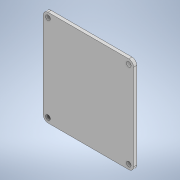
# Autodesk Inventor part: 视孔盖2
Saved by Autodesk Inventor 2020 (Build 240168000, 168)
## iProperties
Created: 2021-06-16
Part Number: 视孔盖2
Material: 常规
Document SubType Name: Modeling
Designer: dell
Density: 1 g/cm^3
Appearance: 默认
Author: dell
Autodesk Inventor part; units mm, degrees
ref_plane "YZ Plane" through (0, 0, 0) normal (1, 0, 0) x (0, 1, 0)
ref_plane "XZ Plane" through (0, 0, 0) normal (0, 1, 0) x (-1, 0, 0)
ref_plane "XY Plane" through (0, 0, 0) normal (0, 0, 1) x (1, 0, 0)
ref_plane "工作平面1" through (0, 0, 0) normal (0, 0, 1) x (1, 0, 0)
sketch "草图1" plane through (0, 0, 0) normal (0, 0, 1) x (1, 0, 0)
  circle A0 centre (-50.5, -54) radius 2.4585 projected
  circle A1 centre (50.5, 54) radius 2.4585 projected
  circle A2 centre (50.5, -54) radius 2.4585 projected
  circle A3 centre (-50.5, 54) radius 2.4585 projected
  arc A4 (56.5, 54) -> (50.5, 60) centre (50.5, 54) ccw projected
  line L0 (50.5, 60) -> (-50.5, 60) projected
  arc A5 (-50.5, 60) -> (-56.5, 54) centre (-50.5, 54) ccw projected
  line L1 (-56.5, 54) -> (-56.5, -54) projected
  arc A6 (-56.5, -54) -> (-50.5, -60) centre (-50.5, -54) ccw projected
  line L2 (-50.5, -60) -> (50.5, -60) projected
  arc A7 (50.5, -60) -> (56.5, -54) centre (50.5, -54) ccw projected
  line L3 (56.5, -54) -> (56.5, 54) projected
  line L4 (-40, -50) -> (-40, 50) construction
  line L5 (-40, 50) -> (40, 50) construction
  line L6 (40, 50) -> (40, -50) construction
  line L7 (40, -50) -> (-40, -50) construction
  point P0 (0, 0)
extrude "拉伸1" add sketch "草图1" along normal blind 4
sketch "草图2" plane through (0, 0, 4) normal (0, 0, 1) x (1, 0, 0)
  circle A0 centre (50.5, 54) radius 2.4585 construction
  circle A1 centre (-50.5, 54) radius 2.4585 construction
  circle A2 centre (-50.5, -54) radius 2.4585 construction
  circle A3 centre (50.5, -54) radius 2.4585 construction
  circle A4 centre (50.5, 54) radius 2.9585
  circle A5 centre (50.5, -54) radius 2.9585
  circle A6 centre (-50.5, 54) radius 2.9585
  circle A7 centre (-50.5, -54) radius 2.9585
  point P0 (0, 0)
  dimension "d2" = 0.5
  dimension "d3" = 0.5
  dimension "d4" = 0.5
  dimension "d5" = 0.5
  constraints: 4 centre point
  measures "d2" radial gap between concentric circles of A0 A4
  measures "d3" radial gap between concentric circles of A3 A5
  measures "d4" radial gap between concentric circles of A1 A6
  measures "d5" radial gap between concentric circles of A2 A7
extrude "拉伸2" cut sketch "草图2" against normal up to surface (4 mm away)
